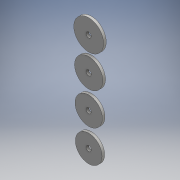
# Autodesk Inventor part: CouplingHeadSilicone_Spacer_3mm
Saved by Autodesk Inventor 2016 (Build 200138000, 138)
## iProperties
Created: 2015-12-22
Part Number: CouplingHeadSilicone_Spacer_3mm
Material: Generic
Document SubType Name: Modeling
Designer: DonMo
Density: 1 g/cm^3
Appearance: Default
Author: DonMo
Autodesk Inventor part; units mm, degrees
ref_plane "YZ Plane" through (0, 0, 0) normal (1, 0, 0) x (0, 1, 0)
ref_plane "XZ Plane" through (0, 0, 0) normal (0, 1, 0) x (-1, 0, 0)
ref_plane "XY Plane" through (0, 0, 0) normal (0, 0, 1) x (1, 0, 0)
sketch "Sketch1" plane through (0, 0, 0) normal (0, 1, 0) x (-1, 0, 0)
  circle A0 centre (0, 0) radius 3.175
  circle A1 centre (0, 0) radius 18.2002
  circle A2 centre (0, -40) radius 3.175
  circle A3 centre (0, -40) radius 17.2423
  circle A4 centre (0, -80) radius 3.175
  circle A5 centre (0, -80) radius 16.6676
  circle A6 centre (0, -120) radius 3.175
  circle A7 centre (0, -120) radius 16.2844
  dimension "d6" = 6.35
  dimension "d10" = 36.4005
  dimension "d24" = 6.35
  dimension "d25" = 34.4847
  dimension "d27" = 6.35
  dimension "d29" = 33.3352
  dimension "d35" = 6.35
  dimension "d36" = 32.5689
  dimension "d43" = 40
  dimension "d44" = 40
  dimension "d45" = 40
  constraints: 8 centre point, 5 coincident, 3 vertical alignment
  measures "d6" diameter of A0
  measures "d10" diameter of A1
  measures "d24" diameter of A2
  measures "d25" diameter of A3
  measures "d27" diameter of A4
  measures "d29" diameter of A5
  measures "d35" diameter of A6
  measures "d36" diameter of A7
  measures "d43" distance of A2.centre point (0, 0)
  measures "d44" distance of A4.centre A2.centre
  measures "d45" distance of A6.centre A4.centre
extrude "Extrusion1" add sketch "Sketch1" along normal blind 3.195
equation "\"d10\" = 0.85 * d1"
equation "\"d25\" = 0.85 * d18"
equation "\"d29\" = 0.85 * d20"
equation "\"d36\" = 0.85 * d22"
equation "\"d46\" = 0.5 * WoodThickness"
equation "\"d1\" = 42.8241"
equation "\"d18\" = 40.5702"
equation "\"d20\" = 39.21786"
equation "\"d22\" = 38.3163"
equation "\"WoodThickness\" = 6.39"
body "Solid1"
